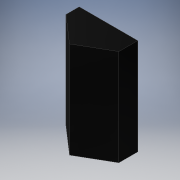
# Autodesk Inventor part: MirrorMountTest
Saved by Autodesk Inventor 2017 (Build 210142000, 142)
## iProperties
Created: 2019-02-22
Part Number: MirrorMountTest
Material: Generic
Document SubType Name: Modeling
Designer: cresswnd
Density: 1 g/cm^3
Appearance: Glossy - Black
Author: cresswnd
Autodesk Inventor part; units mm, degrees
ref_plane "YZ Plane" through (0, 0, 0) normal (1, 0, 0) x (0, 1, 0)
ref_plane "XZ Plane" through (0, 0, 0) normal (0, 1, 0) x (-1, 0, 0)
ref_plane "XY Plane" through (0, 0, 0) normal (0, 0, 1) x (1, 0, 0)
sketch "Sketch1" plane through (0, 0, 0) normal (0, 0, 1) x (1, 0, 0)
  line L0 (0, 0) -> (12.9904, 7.5) construction
  line L1 (0, 0) -> (15, 0) construction
  line L2 (0, 0) -> (-11.3206, 9.8409) construction
  line L3 (0, 0) -> (15, 0) construction
  line L4 (-11.3206, 9.8409) -> (12.9904, 7.5) construction
  line L5 (-11.3206, 9.8409) -> (0, 0)
  line L6 (0, 0) -> (12.9904, 7.5)
  line L7 (12.9904, 7.5) -> (-11.3206, 9.8409)
  line L8 (-11.3206, 9.8409) -> (12.8169, 9.8409) construction
  line L9 (12.8169, 9.8409) -> (12.9904, 7.5) construction
  dimension "d3" = 15
  dimension "d4" = 30
  dimension "d5" = 15
  dimension "d6" = 139
  dimension "d15" = 24.1376
  constraints: 20 end point, 3 horizontal, 2 collinear, 2 equal length
  measures "d3" distance of L0.start L0.end
  measures "d4" angle of L1 L0
  measures "d5" distance of L0.start L2.end
  measures "d6" angle of L3 L2
  measures "d15" distance of L2.end L8.end
extrude "Extrusion1" add sketch "Sketch1" against normal blind 60
sketch "Sketch4" plane through (0, 0, 0) normal (0, 0, 1) x (1, 0, 0)
  line L0 (-11.3206, 9.8409) -> (12.9904, 7.5) projected
  line L1 (-11.3206, 9.8409) -> (12.9904, 9.8409)
  line L2 (12.9904, 9.8409) -> (12.9904, 7.5)
  point P0 (0, 0)
  constraints: 4 end point, 1 horizontal, 1 perpendicular
extrude "Extrusion4" add sketch "Sketch4" against normal blind 60
sketch "Sketch5" plane through (-11.3206, 9.8409, 0) normal (0, 1, 0) x (1, 0, 0)
  line L0 (24.311, 0) -> (0, 0) projected
  line L1 (24.311, 0) -> (24.311, 60) projected
  line L2 (0, 60) -> (24.311, 60) projected
  line L3 (0, 0) -> (0, 60) projected
  line L4 (0, 0) -> (0, 60) projected
  line L5 (0, 30) -> (12.25, 30)
  line L6 (12.25, 30) -> (12.25, 38.89)
  line L7 (11.3206, 0) -> (11.3206, 60) projected
  line L8 (12.25, 30) -> (21.14, 30) construction
  circle A0 centre (12.25, 38.89) radius 0.95
  line L9 (12.25, 30) -> (12.25, 21.11)
  circle A1 centre (12.25, 21.11) radius 0.95
  dimension "d16" = 12.25
  dimension "d17" = 8.89
  dimension "d18" = 90
  dimension "d19" = 1.9
  dimension "d20" = 8.89
  dimension "d21" = 1.9
  constraints: 8 end point, 2 centre point, 2 coincident, 2 horizontal, 1 midpoint, 1 parallel, 1 perpendicular, 1 vertical
  measures "d16" distance of L5.start L5.end
  measures "d17" distance of L5.end L6.end
  measures "d18" angle of L8 L6
  measures "d19" diameter of A0
  measures "d20" distance of L5.end L9.end
  measures "d21" diameter of A1
extrude "Extrusion5" cut sketch "Sketch5" against normal blind 5 contours A1 L7 | L7 A1 | A0 L7 | L7 A0
sketch "Sketch6" plane through (-11.3206, 9.8409, 0) normal (0, 1, 0) x (1, 0, 0)
  circle A0 centre (12.25, 38.89) radius 0.95 projected
  circle A1 centre (12.25, 21.11) radius 0.95 projected
  line L0 (24.311, 0) -> (0, 0) projected
  line L1 (24.311, 0) -> (24.311, 60) projected
  line L2 (0, 60) -> (24.311, 60) projected
  line L3 (0, 0) -> (0, 60) projected
  line L4 (11.3206, 0) -> (11.3206, 10)
  line L5 (11.3206, 0) -> (11.3206, 60) projected
  line L6 (11.3206, 60) -> (11.3206, 50)
  line L7 (0, 0) -> (0, 60) projected
  line L8 (0, 10) -> (24.311, 10)
  line L9 (0, 50) -> (24.311, 50)
  dimension "d24" = 10
  dimension "d25" = 10
  constraints: 8 end point, 6 point on line, 1 horizontal, 1 perpendicular
  measures "d24" distance of L4.start L4.end
  measures "d25" distance of L5.end L6.end
extrude "Extrusion6" cut sketch "Sketch6" against normal blind 20 contours L9 L3 L2 L5 | L5 L2 L1 L9 | L8 L4 L0 L3 | L1 L0 L4 L8
sketch "Sketch7" plane through (-11.3206, 9.8409, -50) normal (0, 1, 0) x (1, 0, 0)
  line L0 (24.311, 0) -> (0, 0) projected
  line L1 (0, -40) -> (0, 0) projected
  line L2 (0, -40) -> (24.311, -40) projected
  line L3 (24.311, -40) -> (24.311, 0) projected
  circle A0 centre (12.25, -11.11) radius 0.95 projected
  circle A1 centre (12.25, -28.89) radius 0.95 projected
  point P0 (11.3206, -50)
extrude "Extrusion7" add sketch "Sketch7" along normal blind 5.5
body "Solid1"
